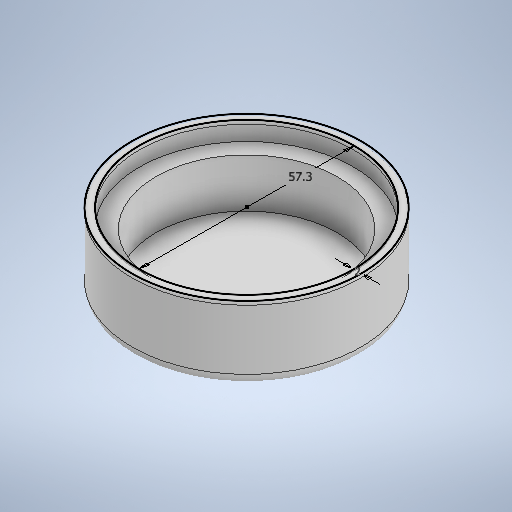
# Autodesk Inventor part: super flash light v4
Saved by Autodesk Inventor 2025 (Build 290162000, 162)
## iProperties
Created: 2024-06-27
Part Number: super flash light v4
Material: 一般
Document SubType Name: Modeling
Designer: gavin
Density: 1 g/cm^3
Appearance: 預設
Author: gavin
## iProperties of the stored document super flash light v4_3D 列印.ipt
Created: 2024-06-27
Part Number: super flash light v4_3D 列印
Material: 一般
Document SubType Name: Modeling
Designer: gavin
Density: 1 g/cm^3
Appearance: 預設
Author: gavin
Autodesk Inventor part; units mm, degrees
ref_plane "YZ Plane" through (0, 0, 0) normal (1, 0, 0) x (0, 1, 0)
ref_plane "XZ Plane" through (0, 0, 0) normal (0, 1, 0) x (-1, 0, 0)
ref_plane "XY Plane" through (0, 0, 0) normal (0, 0, 1) x (1, 0, 0)
sketch "草圖1" plane through (0, 0, 0) normal (0, 1, 0) x (-1, 0, 0)
  circle A0 centre (0, 0) radius 28.65
  circle A1 centre (0, 0) radius 30.65
  dimension "d0" = 57.3
  dimension "d1" = 2
  constraints: 2 centre point, 1 coincident
  measures "d0" diameter of A0
  measures "d1" radial gap between concentric circles of A0 A1
extrude "擠出1" add sketch "草圖1" against normal blind 20 contours A0 | A1
extrude "擠出2" cut sketch "草圖1" against normal blind 5 contours A0
sketch "草圖3" plane through (0, -5, 0) normal (0, 1, 0) x (1, 0, 0)
  circle A0 centre (0, 0) radius 28.65 projected
  circle A1 centre (0, 0) radius 30.65 projected
  circle A2 centre (0, 0) radius 24.25
  dimension "d7" = 4.4
  constraints: 1 centre point
  measures "d7" radial gap between concentric circles of A0 A2
extrude "擠出3" cut sketch "草圖3" against normal blind 13 contours A2
fillet "圓角1" radius 3 1 edges at (30.65, -20, 0)
fillet "圓角2" radius 1 2 edges at (28.65, 0, 0) (30.65, 0, 0)
sketch "草圖4" plane through (0, 0, 0) normal (1, 0, 0) x (0, 1, 0)
  point P0 (0, 0)
